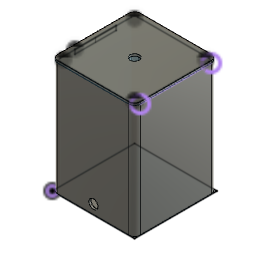
encodeur_btn (Autodesk Fusion 360 design; units mm, degrees)
Autodesk Fusion 360 part; units mm, degrees
sketch "Base" plane through (0, 0, 0) normal (0, 1, 0) x (1, 0, 0) in component "Case"
  line L0 (0, 0) -> (58, 0)
  line L1 (58, 0) -> (58, 58)
  line L2 (58, 58) -> (0, 58)
  line L3 (0, 58) -> (0, 0)
  dimension "d6" = 58
  dimension "d7" = 58
  constraint horizontal L0
  constraint vertical L1
  constraint horizontal L2
  constraint vertical L3
  constraint coincident L0.start L3.end
  measures "d6" distance of L0.start L0.end
  measures "d7" distance of L0.start L2.end
extrude "Extrude1" add sketch "Base" along normal blind 80 makes body 1 in component "Case"
fillet "Fillet1" radius 4 4 edges at (58, 40, 0) (0, 40, 0) (58, 40, -58) (0, 40, -58) on bodies 1 in component "Case"
shell "Shell1" thickness 1.5 removed faces 1 at (18, 80, -19.3333) on bodies 1 in component "Case"
sketch "Knob" plane through (1.5, 0, 0) normal (1, 0, 0) x (0, 0, -1) in component "Case"
  line L0 (54, 1.5) -> (54, 80)
  line L1 (54, 80) -> (4, 80)
  line L2 (4, 80) -> (4, 1.5)
  line L3 (4, 1.5) -> (54, 1.5)
  line L4 (14.5, 80) -> (43.5, 80)
  line L5 (43.5, 80) -> (43.5, 77)
  line L6 (43.5, 77) -> (14.5, 77)
  line L7 (14.5, 77) -> (14.5, 80)
  line L8 (29, 80) -> (29, 77) construction
  dimension "d12" = 29
  dimension "d13" = 3
  constraint horizontal L4
  constraint vertical L5
  constraint horizontal L6
  constraint vertical L7
  constraint coincident L1 L4.start
  constraint midpoint L1 L8.start
  constraint midpoint L6 L8.end
  constraint vertical L8
  measures "d12" distance of L5.end L6.end
  measures "d13" distance of L4.end L5.end
extrude "Extrude2" add sketch "Knob" along normal blind 6 draft -45 contours L1 L4 L5 L6 L7 bodies 1 in component "Case"
ref_plane "WorkPlane2" through (29, 40, -29) normal (-1, 0, 0) x (0, 0, 1) in component "Case"
mirror "Mirror1" about plane through (29, 40, -29) normal (-1, 0, 0) of "Extrude2" in component "Case"
sketch "Top" plane through (0, 80, 0) normal (0, 1, 0) x (-1, 0, 0) in component "Top Cover"
  line L0 (-58, -4) -> (-58, -54)
  arc A0 (-58, -54) -> (-54, -58) centre (-54, -54) ccw
  line L1 (-54, -58) -> (-4, -58)
  arc A1 (-4, -58) -> (0, -54) centre (-4, -54) ccw
  line L2 (0, -54) -> (0, -4)
  arc A2 (0, -4) -> (-4, 0) centre (-4, -4) ccw
  line L3 (-4, 0) -> (-54, 0)
  arc A3 (-54, 0) -> (-58, -4) centre (-54, -4) ccw
  line L4 (-56.5, -14.5) -> (-56.5, -4)
  arc A4 (-54, -1.5) -> (-56.5, -4) centre (-54, -4) ccw
  line L5 (-54, -1.5) -> (-4, -1.5)
  arc A5 (-1.5, -4) -> (-4, -1.5) centre (-4, -4) ccw
  line L6 (-1.5, -4) -> (-1.5, -14.5)
  line L7 (-1.5, -14.5) -> (-1.5, -43.5)
  line L8 (-1.5, -43.5) -> (-1.5, -54)
  arc A6 (-4, -56.5) -> (-1.5, -54) centre (-4, -54) ccw
  line L9 (-4, -56.5) -> (-54, -56.5)
  arc A7 (-56.5, -54) -> (-54, -56.5) centre (-54, -54) ccw
  line L10 (-56.5, -54) -> (-56.5, -43.5)
  line L11 (-56.5, -43.5) -> (-56.5, -14.5)
extrude "Extrude1'" add sketch "Top" along normal blind 1.5 separate body contours L0 A0 L1 A1 L2 A2 L3 A3 | L4 A4 L5 A5 L6 L7 L8 A6 L9 A7 L10 L11 makes body 2 in component "Top Cover"
sketch "Lip" plane through (0, 80, 0) normal (0, -1, 0) x (1, 0, 0) in component "Top Cover"
  arc A0 (58, -4) -> (54, 0) centre (54, -4) ccw
  line L0 (54, 0) -> (4, 0)
  arc A1 (4, 0) -> (0, -4) centre (4, -4) ccw
  line L1 (0, -4) -> (0, -54)
  arc A2 (0, -54) -> (4, -58) centre (4, -54) ccw
  line L2 (4, -58) -> (54, -58)
  arc A3 (54, -58) -> (58, -54) centre (54, -54) ccw
  line L3 (58, -54) -> (58, -4)
  line L4 (56.3, -54) -> (56.3, -4)
  arc A4 (56.3, -4) -> (54, -1.7) centre (54, -4) ccw
  line L5 (54, -1.7) -> (4, -1.7)
  arc A5 (4, -1.7) -> (1.7, -4) centre (4, -4) ccw
  line L6 (1.7, -4) -> (1.7, -54)
  arc A6 (1.7, -54) -> (4, -56.3) centre (4, -54) ccw
  line L7 (4, -56.3) -> (54, -56.3)
  arc A7 (54, -56.3) -> (56.3, -54) centre (54, -54) ccw
  line L8 (58, -4) -> (58, -54)
  dimension "d19" = 1.7
  dimension "d31" = 1.7
  measures "d31" distance of L4 L8
extrude "Extrude2'" add sketch "Lip" along normal blind 3 contours L4 A4 L5 A5 L6 A6 L7 A7 bodies 2 in component "Top Cover"
extrude "Extrude3" cut sketch "Knob" along normal blind 3 draft -45 from surface at 0.2 contours L1 L4 L5 L6 L7 bodies 2 in component "Top Cover"
ref_plane "WorkPlane2" through (29, 0, 0) normal (1, 0, 0) x (0, 1, 0) in component "Top Cover"
mirror "Mirror1'" about plane through (29, 0, 0) normal (1, 0, 0) of "Extrude3" in component "Top Cover"
shell "Shell1'" thickness 1.5 removed faces 1 at (38.1, 77, -33.8333) on bodies 2 in component "Top Cover"
chamfer "Chamfer1" distance 0.6 angle 45 2 edges at (1.7, 77, -29) (56.3, 77, -29) on bodies 2 in component "Top Cover"
sketch "Sketch1" plane through (2.1865, 81.5, -5.8403) normal (0, 1, 0) x (-1, 0, 0)
  line L0 (-55.8135, 1.8403) -> (-55.8135, -48.1597)
  arc A0 (-55.8135, -48.1597) -> (-51.8135, -52.1597) centre (-51.8135, -48.1597) ccw
  line L1 (-51.8135, -52.1597) -> (-1.8135, -52.1597)
  arc A1 (-1.8135, -52.1597) -> (2.1865, -48.1597) centre (-1.8135, -48.1597) ccw
  line L2 (2.1865, -48.1597) -> (2.1865, 1.8403)
  arc A2 (2.1865, 1.8403) -> (-1.8135, 5.8403) centre (-1.8135, 1.8403) ccw
  line L3 (-1.8135, 5.8403) -> (-51.8135, 5.8403)
  arc A3 (-51.8135, 5.8403) -> (-55.8135, 1.8403) centre (-51.8135, 1.8403) ccw
  circle A4 centre (-26.8135, -23.1597) radius 3.25
  dimension "d36" = 6.5
  dimension "d37" = 29
  dimension "d38" = 29
  measures "d36" diameter of A4
  measures "d37" distance of L2 A4.centre
  measures "d38" distance of L3 A4.centre
hole "Hole1" at (29, 81.5, -29) direction (0, -1, 0) diameter 6.5 depth 10 tip angle 180 bodies 2 in component "Top Cover"
sketch "Sketch2" plane through (0, 0, -58) normal (0, 0, -1) x (-1, 0, 0)
  line L0 (-4, 0) -> (-4, 80)
  line L1 (-4, 80) -> (-54, 80)
  line L2 (-54, 80) -> (-54, 0)
  line L3 (-54, 0) -> (-4, 0)
  line L4 (-35, 47.5) -> (-23, 47.5)
  line L5 (-23, 47.5) -> (-23, 35.5)
  line L6 (-23, 35.5) -> (-35, 35.5)
  line L7 (-35, 35.5) -> (-35, 47.5)
  line L8 (0, 0) -> (0, 80)
  line L9 (-54, 81.5) -> (-4, 81.5)
  dimension "d42" = 12
  dimension "d43" = 12
  dimension "d45" = 23
  dimension "d46" = 34
  constraint horizontal L4
  constraint vertical L5
  constraint horizontal L6
  constraint vertical L7
  measures "d42" distance of L4.start L4.end
  measures "d43" distance of L4.start L6.end
  measures "d45" distance of L5 L8
  measures "d46" distance of L4 L9
extrude "Extrude3'" cut sketch "Sketch2" against normal blind 10 contours L4 L5 L6 L7 bodies 1 in component "Case"
sketch "Sketch3" plane through (0, 0, 0) normal (0, 0, 1) x (1, 0, 0)
  line L0 (4, 80) -> (4, 0)
  line L1 (4, 0) -> (54, 0)
  line L2 (54, 0) -> (54, 80)
  line L3 (54, 80) -> (4, 80)
  circle A0 centre (29, 6.5) radius 3
  line L4 (58, 0) -> (58, 80)
  line L5 (0, 0) -> (58, 0)
  dimension "d49" = 6
  dimension "d50" = 29
  dimension "d51" = 6.5
  measures "d49" diameter of A0
  measures "d50" distance of A0.centre L4
  measures "d51" distance of A0.centre L5
hole "Hole1'" at (29, 6.5, 0) direction (0, 0, -1) diameter 6.5 depth 10 tip angle 180 bodies 1 in component "Case"
component "Enclosure" placed x (1, 0, 0) y (0, 1, 0) z (0, 0, 1) at (0, 0, 0)
component "Case" placed x (1, 0, 0) y (0, 1, 0) z (0, 0, 1) at (0, 0, 0) in component "Enclosure"
component "Top Cover" placed x (1, 0, 0) y (0, 1, 0) z (0, 0, 1) at (0, 0, 0) in component "Enclosure"
equation "Width = Width_internal + ( 2 * shell )"
equation "length = Length_internal + ( 2 * shell )"
equation "heigth = 80 mm"
equation "shell = 1.5 mm"
equation "gap = 0.2 mm"
equation "d6 = length"
equation "d7 = Width"
equation "d8 = heigth"
equation "d11 = shell"
equation "d12 = Width / 2"
equation "d13 = shell * 2"
equation "d17 = shell"
equation "d19 = shell + gap"
equation "d20 = shell * 2"
equation "d23 = shell * 2"
equation "d26 = shell"
equation "d31 = shell + gap"
equation "d33 = length / 2"
equation "Width_internal = 55 mm"
equation "Length_internal = 55 mm"
equation "d37 = Width / 2"
equation "d38 = Width / 2"
equation "d45 = Width / 2 - 6 mm"
equation "d46 = heigth / 2 - 6 mm"
equation "d50 = Width / 2"
equation "d51 = shell + 5 mm"
